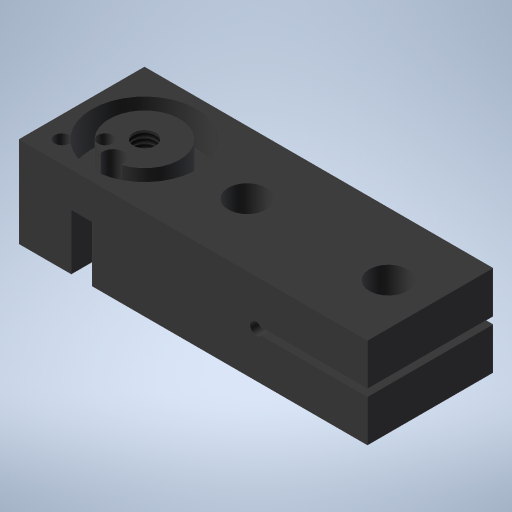
# Autodesk Inventor part: levelmeter-top
Saved by Autodesk Inventor 2024 (Build 280153000, 153)
## iProperties
Created: 2023-09-12
Part Number: levelmeter-top
Material: Generic
Document SubType Name: Modeling
Designer: raad
Density: 1 g/cm^3
Appearance: Default
Author: raad
Autodesk Inventor part; units mm, degrees
ref_plane "YZ Plane" through (0, 0, 0) normal (1, 0, 0) x (0, 1, 0)
ref_plane "XZ Plane" through (0, 0, 0) normal (0, 1, 0) x (-1, 0, 0)
ref_plane "XY Plane" through (0, 0, 0) normal (0, 0, 1) x (1, 0, 0)
sketch "Sketch1" plane through (0, 0, 0) normal (0, 0, 1) x (1, 0, 0)
  line L0 (-25, -6.5) -> (25, -6.5)
  line L1 (25, -6.5) -> (25, 6.5)
  line L2 (25, 6.5) -> (-25, 6.5)
  line L3 (-25, 6.5) -> (-25, -6.5)
  line L4 (-25, -6.5) -> (25, 6.5) construction
  line L5 (25, -6.5) -> (-25, 6.5) construction
  line L6 (25, 0) -> (9, 0)
  circle A0 centre (9, 0) radius 0.89
  line L7 (25, 0) -> (25, 0.5)
  line L8 (25, 0.5) -> (9.7363, 0.5)
  line L9 (25, 0) -> (25, -0.5)
  line L10 (25, -0.5) -> (9.7363, -0.5)
  point P0 (0, 0)
  dimension "d0" = 50
  dimension "d1" = 13
  dimension "d2" = 16
  dimension "d3" = 1.78
  dimension "d4" = 0.5
  dimension "d5" = 0.5
  constraints: 22 end point, 3 midpoint, 3 perpendicular, 2 horizontal, 2 parallel, 2 point on circle, 2 point on line, 1 centre point, 1 coincident
  measures "d0" distance of L2.end L1.end
  measures "d1" distance of L1.end L0.end
  measures "d2" distance of L6.start L6.end
  measures "d3" diameter of A0
  measures "d4" distance of L6.start L7.end
  measures "d5" distance of L6.start L9.end
extrude "Extrusion1" add sketch "Sketch1" against normal blind 18 contours L3 L2 L1 L8 A0 L10 L0
sketch "Sketch2" plane through (-25, -6.5, 0) normal (0, -1, 0) x (1, 0, 0)
  line L0 (50, 0) -> (50, -18) projected
  line L1 (50, -9) -> (44, -9)
  line L2 (44, -9) -> (23.75, -9)
  circle A0 centre (44, -9) radius 4.375
  circle A1 centre (23.75, -9) radius 4.375
  line L3 (0, 0) -> (7.5, 0)
  line L4 (50, 0) -> (0, 0) projected
  line L5 (7.5, 0) -> (9, 0)
  line L6 (9, 0) -> (9, -5)
  circle A2 centre (9, -5) radius 1.5
  line L7 (7.5, 0) -> (7.5, -5)
  line L8 (9, 0) -> (10.5, 0)
  line L9 (10.5, 0) -> (10.5, -5)
  point P0 (25, 0)
  dimension "d8" = 6
  dimension "d9" = 20.25
  dimension "d10" = 8.75
  dimension "d11" = 8.75
  dimension "d12" = 7.5
  dimension "d13" = 1.5
  dimension "d14" = 5
  dimension "d15" = 3
  constraints: 16 end point, 4 point on line, 3 centre point, 3 coincident, 2 point on circle, 1 horizontal, 1 midpoint, 1 perpendicular, 1 tangent, 1 vertical
  measures "d8" distance of L1.start L1.end
  measures "d9" distance of L1.end L2.end
  measures "d10" diameter of A0
  measures "d11" diameter of A1
  measures "d12" distance of L3.start L3.end
  measures "d13" distance of L3.end L5.end
  measures "d14" distance of L5.end L6.end
  measures "d15" diameter of A2
hole "Hole1" at (19, -6.5, -9) at (-1.25, -6.5, -9) direction (0, 1, 0) diameter 5.5 end through all clearance for "Socket Head Cap Screw ISO 4762" size "M5" standard "ISO"
extrude "Extrusion2" cut sketch "Sketch2" against normal blind 8 contours L9 A2 L6 L4 | L6 A2 L7 L4 | A2
sketch "Sketch3" plane through (-25, 6.5, 0) normal (0, 1, 0) x (1, 0, 0)
  line L0 (0, 0) -> (0, 18) projected
  line L1 (0, 0) -> (18, 18)
  line L2 (0, 18) -> (50, 18) projected
  line L3 (0, 0) -> (25.4558, 0) construction
  circle A0 centre (9, 9) radius 7.55
  circle A1 centre (9, 9) radius 5.05
  circle A2 centre (9, 9) radius 2
  line L4 (9, 7) -> (9, 4.5)
  circle A3 centre (9, 4.5) radius 1.5
  line L5 (5.4291, 5.4291) -> (6.1857, 6.1857)
  circle A4 centre (6.1857, 6.1857) radius 1.085
  line L6 (0, 0) -> (3.085, 3.085)
  circle A5 centre (3.085, 3.085) radius 1.085
  point P0 (25, 0)
  point P1 (4.1636, 3.2024)
  point P2 (3.2024, 4.1636)
  point P3 (7.5376, 4.1664)
  point P4 (5.5752, 5.2888)
  point P5 (5.2888, 5.5752)
  point P6 (10.4624, 4.1664)
  dimension "d27" = 10.1
  dimension "d28" = 4
  dimension "d25" = 45
  dimension "d26" = 15.1
  dimension "d29" = 2.5
  dimension "d30" = 3
  dimension "d31" = 1.07
  dimension "d32" = 2.17
  dimension "d33" = 4.3628
  dimension "d34" = 2.17
  constraints: 10 end point, 5 coincident, 4 centre point, 4 point on line, 1 equal length, 1 horizontal, 1 midpoint, 1 vertical, 1 vertical alignment, 5 other
  measures "d25" angle of L3 L1
  measures "d26" diameter of A0
  measures "d29" distance of L4.start L4.end
  measures "d30" diameter of A3
  measures "d31" distance of L5.start L5.end
  measures "d32" diameter of A4
  measures "d33" distance of L0.start L6.end
  measures "d34" diameter of A5
extrude "Extrusion3" cut sketch "Sketch3" against normal blind 5 contours A0 L1 A1 A4 A5 | A0 A5 L1 A4 A1 A3 | A3 A1 | A1 A3
hole "Hole2" at (-16, 6.5, -9) direction (0, -1, 0) diameter 3.242 depth 8.5 tip angle 118 thread size "M4x0.7" class "6H" standard "ISO Metric profile"
hole "Hole3" at (-18.8143, 6.5, -6.1857) at (-21.915, 6.5, -3.085) direction (0, -1, 0) diameter 2.17 depth 8.5
body "Solid1"
